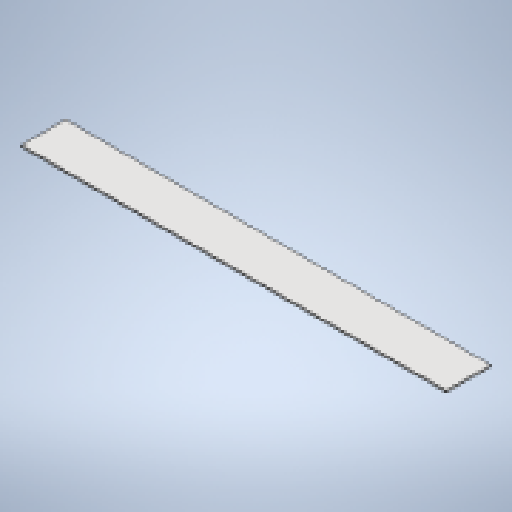
# Autodesk Inventor part: TRM 024 top damper
Saved by Autodesk Inventor 2025.1 (Build 291241020, 241B)
## iProperties
Created: 2024-08-07
Part Number: TRM 024 top damper
Material: AISI 304
Document SubType Name: Sheet Metal
Designer: pokla
Density: 8.02768 g/cm^3
Flat Pattern Width: 48 cm
Flat Pattern Length: 7.46839 cm
Flat Pattern Area: 358.483 cm^2
Sheet Metal Rule: AISI304 2mm Die16
Sheet Metal Width: 480.000 mm
Sheet Metal Length: 74.684 mm
Sheet Metal Area: 35848.261 mm^2
Appearance: Default
Stock Number: ТРМ 024 верх успокоитель
Author: pokla
Autodesk Inventor part; units mm, degrees
ref_plane "YZ Plane" through (0, 0, 0) normal (1, 0, 0) x (0, 1, 0)
ref_plane "XZ Plane" through (0, 0, 0) normal (0, 1, 0) x (-1, 0, 0)
ref_plane "XY Plane" through (0, 0, 0) normal (0, 0, 1) x (1, 0, 0)
sketch "Sketch1" plane through (0, 0, 0) normal (0, 0, 1) x (1, 0, 0)
  line L0 (-240, -15) -> (240, -15)
  line L1 (240, -15) -> (240, 15)
  line L2 (240, 15) -> (-240, 15)
  line L3 (-240, 15) -> (-240, -15)
  line L4 (-240, -15) -> (240, 15) construction
  line L5 (240, -15) -> (-240, 15) construction
  point P0 (0, 0)
  dimension "d0" = 480
  dimension "d1" = 30
  measures "d0" distance of L2.end L1.end
  measures "d1" distance of L1.end L0.end
extrude "Plate1" add sketch "Sketch1" along normal blind 2
sketch "Sketch2" plane through (0, 0, 0) normal (0, 0, -1) x (-1, 0, 0)
  line L0 (-220, 5) -> (-20, 5) construction
  line L1 (-20, 5) -> (-20, -15) construction
  line L2 (-20, -15) -> (-220, -15) construction
  line L3 (-220, -15) -> (-220, 5) construction
  line L4 (-240, 15) -> (240, 15) projected
  line L5 (-240, -15) -> (-240, 15) projected
  point P0 (0, 0)
  dimension "d6" = 200
  dimension "d9" = 20
  dimension "d10" = 10
  dimension "d11" = 20
  constraints: 2 other
  measures "d6" distance of L0.start L0.end
  measures "d9" distance of L0.end L1.end
  measures "d10" distance between parallel lines of L4 L0
  measures "d11" distance between parallel lines of L5 L3
mark "Mark1"
sketch "Sketch3" plane through (240, -13.0049, -0.1395) normal (0, -0.9975641, 0.0697565) x (1, 0, 0)
  line L0 (-480, 0) -> (0, 0)
  line L1 (0, 0) -> (0, 25)
  line L2 (0, 25) -> (-480, 25)
  line L3 (-480, 25) -> (-480, 0)
  constraints: 6 end point, 1 horizontal, 1 perpendicular, 1 vertical
edge flange "Flange1" height 25 angle 94 thickness 2 bend radius 2.75 thickness toward (0, -0.9975641, 0.0697565) relief round relief width 2 relief depth 1 edges at (0, -15, 2) wall of the first edge with corners at (-240, -13.0049, -0.1395) (240, -13.0049, -0.1395) (240, -11.261, 24.7996) (-240, -11.261, 24.7996)
bend "Bend1"
corner "Corner1"
sketch "Sketch4" plane through (-240, 13.5858, 1.4142) normal (0, 0.7071068, -0.7071068) x (-1, 0, 0)
  line L0 (-480, 0) -> (0, 0)
  line L1 (0, 0) -> (0, 25)
  line L2 (0, 25) -> (-480, 25)
  line L3 (-480, 25) -> (-480, 0)
  constraints: 6 end point, 1 horizontal, 1 perpendicular, 1 vertical
edge flange "Flange2" height 25 angle 45 thickness 2 bend radius 2.75 thickness toward (0, 0.7071068, -0.7071068) relief round relief width 2 relief depth 1 edges at (0, 15, 2) wall of the first edge with corners at (240, 13.5858, 1.4142) (-240, 13.5858, 1.4142) (-240, 31.2635, 19.0919) (240, 31.2635, 19.0919)
bend "Bend2"
corner "Corner2"
equation "\"d2\" = Thickness"
equation "\"d12\" = BendReliefWidth"
equation "\"d13\" = BendReliefDepth"
equation "\"d14\" = MinimumRemnant"
equation "\"d15\" = TransitionRadius"
equation "\"d18\" = BendRadius"
equation "\"d19\" = CornerReliefSize"
equation "\"d20\" = GapSize"
equation "\"d21\" = JacobiRadiusSize"
equation "\"d22\" = BendReliefWidth"
equation "\"d23\" = BendReliefDepth"
equation "\"d24\" = MinimumRemnant"
equation "\"d25\" = TransitionRadius"
equation "\"d28\" = BendRadius"
equation "\"d29\" = CornerReliefSize"
equation "\"d30\" = GapSize"
equation "\"d31\" = JacobiRadiusSize"
equation "\"BendReliefWidth\" = Thickness"
equation "\"BendReliefDepth\" = 0.5 * Thickness"
equation "\"CornerReliefSize\" = 4 * Thickness"
equation "\"MinimumRemnant\" = 2 * Thickness"
equation "\"TransitionRadius\" = BendRadius"
equation "\"JacobiRadiusSize\" = BendRadius"
equation "\"GapSize\" = Thickness"
equation "\"Thickness\" = 2"
equation "\"BendRadius\" = 2.75"
body "Solid1"
